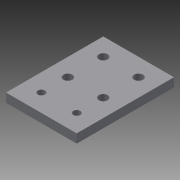
# Autodesk Inventor part: CatapultPlate
Saved by Autodesk Inventor 2013 (Build 170138000, 138)
## iProperties
Created: 2014-01-18
Part Number: CatapultPlate
Material: Generic
Document SubType Name: Modeling
Designer: 215152
Density: 1 g/cm^3
Author: 215152
Autodesk Inventor part; units mm, degrees
ref_plane "YZ Plane" through (0, 0, 0) normal (1, 0, 0) x (0, 1, 0)
ref_plane "XZ Plane" through (0, 0, 0) normal (0, 1, 0) x (-1, 0, 0)
ref_plane "XY Plane" through (0, 0, 0) normal (0, 0, 1) x (1, 0, 0)
sketch "Sketch1" plane through (0, 0, 0) normal (0, 1, 0) x (-1, 0, 0)
  line L0 (25.4, 34.925) -> (-25.4, 34.925)
  line L1 (-25.4, 34.925) -> (-25.4, -34.925)
  line L2 (-25.4, -34.925) -> (25.4, -34.925)
  line L3 (25.4, -34.925) -> (25.4, 34.925)
  line L4 (25.4, 34.925) -> (-25.4, -34.925) construction
  line L5 (-25.4, 34.925) -> (25.4, -34.925) construction
  line L6 (25.4, -34.925) -> (12.7, -34.925)
  line L7 (25.4, -22.225) -> (25.4, -34.925)
  line L8 (-25.4, -34.925) -> (-12.7, -34.925)
  line L9 (-12.7, -22.225) -> (-25.4, -22.225)
  line L10 (-25.4, -22.225) -> (-25.4, -34.925)
  line L11 (12.7, -22.225) -> (12.7, 3.175)
  line L12 (12.7, -22.225) -> (38.1, -22.225) construction
  line L13 (-12.7, -22.225) -> (-12.7, 3.175)
  line L14 (25.4, 34.925) -> (12.7, 34.925)
  line L15 (25.4, 22.225) -> (25.4, 34.925)
  line L16 (-25.4, 34.925) -> (-12.7, 34.925)
  line L17 (-25.4, 22.225) -> (-25.4, 34.925)
  circle A0 centre (12.7, 22.225) radius 2.54
  circle A1 centre (-12.7, 22.225) radius 2.54
  circle A2 centre (12.7, -22.225) radius 3.175
  circle A3 centre (-12.7, -22.225) radius 3.175
  circle A4 centre (12.7, 3.175) radius 3.175
  circle A5 centre (-12.7, 3.175) radius 3.175
  point P0 (0, 0)
  dimension "d0" = 50.8
  dimension "d1" = 69.85
  dimension "d2" = 12.7
  dimension "d3" = 12.7
  dimension "d4" = 12.7
  dimension "d5" = 12.7
  dimension "d6" = 25.4
  dimension "d7" = 90
  dimension "d8" = 25.4
  dimension "d13" = 5.08
  dimension "d14" = 5.08
  dimension "d15" = 6.35
  dimension "d16" = 6.35
  dimension "d17" = 6.35
  dimension "d18" = 6.35
  constraints: 36 end point, 6 centre point, 6 horizontal, 4 coincident, 4 parallel, 3 perpendicular, 2 midpoint
  measures "d0" distance of L2.end L1.end
  measures "d1" distance of L1.end L0.end
  measures "d2" distance of L11.start L7.start
  measures "d3" distance of L6.end L11.start
  measures "d4" distance of L9.end L9.start
  measures "d5" distance of L9.start L8.end
  measures "d6" distance of L11.start L11.end
  measures "d7" angle of L12 L11
  measures "d8" distance of L9.start L13.end
  measures "d13" diameter of A0
  measures "d14" diameter of A1
  measures "d15" diameter of A2
  measures "d16" diameter of A3
  measures "d17" diameter of A4
  measures "d18" diameter of A5
extrude "Extrusion1" add sketch "Sketch1" along normal blind 6.35
body "Solid1"
